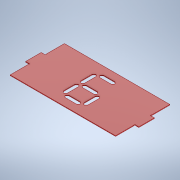
# Autodesk Inventor part: Cockpit_front_frame_cloth
Saved by Autodesk Inventor 2020.4 (Build 244396000, 396)
## iProperties
Created: 2022-04-01
Part Number: Cockpit_front_frame_cloth
Material: 一般
Document SubType Name: Modeling
Designer: Masato Kubotera
Density: 1 g/cm^3
Appearance: 滑らか - 赤
Author: Masato Kubotera
Autodesk Inventor part; units mm, degrees
ref_plane "XZ Plane" through (0, 0, 0) normal (0, 1, 0) x (-1, 0, 0)
ref_plane "XY Plane" through (0, 0, 0) normal (0, 0, 1) x (1, 0, 0)
derived "Cockpit_front_frame.ipt"
sketch "スケッチ2" plane through (0, 0, 0) normal (0, 1, 0) x (-1, 0, 0)
  line L0 (-28.5, -22.5) -> (88.5, -22.5) construction
  line L1 (88.5, -22.5) -> (88.5, -138.5)
  line L2 (88.5, -96) -> (-28.5, -96) construction
  line L3 (-28.5, -96) -> (-28.5, -22.5) construction
  line L4 (-28.5, -22.5) -> (88.5, -96) construction
  line L5 (88.5, -22.5) -> (-28.5, -96) construction
  line L6 (38.5, -101) -> (38.5, -133.5)
  line L7 (43.5, -138.5) -> (88.5, -138.5)
  line L8 (63.9, -63.85) -> (73.1, -63.85) construction
  line L9 (73.1, -63.85) -> (73.1, -77.65) construction
  line L10 (73.1, -77.65) -> (63.9, -77.65) construction
  line L11 (63.9, -77.65) -> (63.9, -63.85) construction
  line L12 (63.9, -63.85) -> (73.1, -77.65) construction
  line L13 (73.1, -63.85) -> (63.9, -77.65) construction
  line L14 (63.2, -63.2) -> (73.8, -63.2) construction
  line L15 (73.8, -63.2) -> (73.8, -78.3) construction
  line L16 (73.8, -78.3) -> (63.2, -78.3) construction
  line L17 (63.2, -78.3) -> (63.2, -63.2) construction
  line L18 (63.2, -63.2) -> (73.8, -78.3) construction
  line L19 (73.8, -63.2) -> (63.2, -78.3) construction
  line L20 (68.5, -63.2) -> (68.5, -78.3) construction
  line L21 (73.8, -70.75) -> (63.2, -70.75) construction
  line L22 (64.6349, -63.15) -> (72.3651, -63.15)
  line L23 (63.15, -64.6349) -> (63.15, -76.8651)
  line L24 (65.3349, -63.8) -> (71.6651, -63.8)
  line L25 (63.85, -65.2849) -> (63.85, -76.2151)
  arc A0 (64.6349, -63.15) -> (63.15, -64.6349) centre (63.8925, -63.8925) ccw
  arc A1 (65.3349, -63.8) -> (63.85, -65.2849) centre (64.5925, -64.5425) ccw
  arc A2 (73.85, -64.6349) -> (72.3651, -63.15) centre (73.1075, -63.8925) ccw
  arc A3 (73.15, -65.2849) -> (71.6651, -63.8) centre (72.4075, -64.5425) ccw
  line L26 (64.6349, -78.35) -> (72.3651, -78.35)
  line L27 (65.3349, -77.7) -> (71.6651, -77.7)
  arc A4 (63.85, -76.2151) -> (65.3349, -77.7) centre (64.5925, -76.9575) ccw
  arc A5 (63.15, -76.8651) -> (64.6349, -78.35) centre (63.8925, -77.6075) ccw
  arc A6 (72.3651, -78.35) -> (73.85, -76.8651) centre (73.1075, -77.6075) ccw
  arc A7 (71.6651, -77.7) -> (73.15, -76.2151) centre (72.4075, -76.9575) ccw
  line L28 (73.15, -65.2849) -> (73.15, -76.2151)
  line L29 (73.85, -64.6349) -> (73.85, -76.8651)
  line L30 (-23.5, -22.5) -> (-28.5, -27.5)
  line L31 (-28.5, -59.25) -> (88.5, -59.25) construction
  line L32 (30, -22.5) -> (30, -96) construction
  line L33 (-23.5, -96) -> (-28.5, -91)
  line L34 (-28.5, -27.5) -> (-28.5, -91)
  line L35 (-20.5, -24.5) -> (-25.5, -24.5) construction
  line L36 (-25.5, -24.5) -> (-25.5, -94) construction
  line L37 (-25.5, -94) -> (-20.5, -94) construction
  line L38 (-20.5, -94) -> (-20.5, -24.5) construction
  line L39 (-20.5, -24.5) -> (-25.5, -94) construction
  line L40 (-25.5, -24.5) -> (-20.5, -94) construction
  line L41 (-25.55, -46.7) -> (-20.45, -46.7)
  line L42 (-20.45, -46.7) -> (-20.45, -71.8)
  line L43 (-20.45, -71.8) -> (-25.55, -71.8)
  line L44 (-25.55, -71.8) -> (-25.55, -46.7)
  line L45 (-25.55, -46.7) -> (-20.45, -71.8) construction
  line L46 (-20.45, -46.7) -> (-25.55, -71.8) construction
  line L47 (-25.5, -46.75) -> (-20.5, -46.75) construction
  line L48 (-25.5, -71.75) -> (-20.5, -71.75) construction
  line L49 (-23, -24.5) -> (-23, -94) construction
  circle A8 centre (-23, -35) radius 3
  circle A9 centre (-23, -35) radius 1.6
  arc A10 (-24.0651, -46.7) -> (-25.55, -48.1849) centre (-24.8075, -47.4425) ccw
  arc A11 (-20.45, -48.1849) -> (-21.9349, -46.7) centre (-21.1925, -47.4425) ccw
  arc A12 (-25.55, -70.3151) -> (-24.0651, -71.8) centre (-24.8075, -71.0575) ccw
  arc A13 (-21.9349, -71.8) -> (-20.45, -70.3151) centre (-21.1925, -71.0575) ccw
  circle A14 centre (-23, -83.5) radius 3
  circle A15 centre (-23, -83.5) radius 1.6
  line L50 (33.5, -96) -> (38.5, -101)
  line L51 (-23.5, -96) -> (33.5, -96)
  line L52 (81, -46.5) -> (-20.5, -46.5) construction
  line L53 (-20.5, -46.5) -> (-20.5, -41.5) construction
  line L54 (-20.5, -41.5) -> (81, -41.5) construction
  line L55 (81, -41.5) -> (81, -46.5) construction
  line L56 (81, -46.5) -> (-20.5, -41.5) construction
  line L57 (-20.5, -46.5) -> (81, -41.5) construction
  line L58 (-20.5, -44) -> (81, -44) construction
  line L59 (30.25, -41.5) -> (30.25, -46.5) construction
  line L60 (5.25, -41.5) -> (5.25, -46.5) construction
  line L61 (55.3, -41.45) -> (5.2, -41.45)
  line L62 (5.2, -41.45) -> (5.2, -46.55)
  line L63 (5.2, -46.55) -> (55.3, -46.55)
  line L64 (55.3, -46.55) -> (55.3, -41.45)
  line L65 (55.3, -41.45) -> (5.2, -46.55) construction
  line L66 (5.2, -41.45) -> (55.3, -46.55) construction
  arc A16 (6.6849, -41.45) -> (5.2, -42.9349) centre (5.9425, -42.1925) ccw
  circle A17 centre (-2.25, -44) radius 3
  circle A18 centre (-2.25, -44) radius 1.6
  line L67 (55.25, -41.5) -> (55.25, -46.5) construction
  arc A19 (55.3, -42.9349) -> (53.8151, -41.45) centre (54.5575, -42.1925) ccw
  circle A20 centre (62.75, -44) radius 3
  circle A21 centre (62.75, -44) radius 1.6
  arc A22 (5.2, -45.0651) -> (6.6849, -46.55) centre (5.9425, -45.8075) ccw
  arc A23 (53.8151, -46.55) -> (55.3, -45.0651) centre (54.5575, -45.8075) ccw
  line L68 (-20.5, -89) -> (81, -89) construction
  line L69 (81, -89) -> (81, -94) construction
  line L70 (81, -94) -> (-20.5, -94) construction
  line L71 (-20.5, -94) -> (-20.5, -89) construction
  line L72 (-20.5, -89) -> (81, -94) construction
  line L73 (81, -89) -> (-20.5, -94) construction
  line L74 (-20.5, -91.5) -> (81, -91.5) construction
  line L75 (30.25, -89) -> (30.25, -94) construction
  line L76 (55.3, -91.55) -> (5.2, -91.55)
  line L77 (5.2, -91.55) -> (5.2, -88.95)
  line L78 (5.2, -88.95) -> (55.3, -88.95)
  line L79 (55.3, -88.95) -> (55.3, -91.55)
  line L80 (55.3, -91.55) -> (5.2, -88.95) construction
  line L81 (5.2, -91.55) -> (55.3, -88.95) construction
  line L82 (5.25, -89) -> (5.25, -91.5) construction
  line L83 (55.25, -89) -> (55.25, -91.5) construction
  line L84 (5.25, -90.25) -> (55.25, -90.25) construction
  arc A24 (7.3, -88.95) -> (5.2, -88.95) centre (6.25, -88.95) ccw
  arc A25 (55.3, -88.95) -> (53.2, -88.95) centre (54.25, -88.95) ccw
  arc A26 (5.2, -91.55) -> (7.3, -91.55) centre (6.25, -91.55) ccw
  arc A27 (53.2, -91.55) -> (55.3, -91.55) centre (54.25, -91.55) ccw
  circle A28 centre (-2.5, -91.5) radius 3
  circle A29 centre (-2.5, -91.5) radius 1.6
  circle A30 centre (62.5, -91.5) radius 3 construction
  circle A31 centre (62.5, -91.5) radius 1.6 construction
  line L85 (-23.5, -22.5) -> (63.7651, -22.5)
  line L86 (65.25, -21.0151) -> (65.25, -17.5)
  line L87 (65.25, -17.5) -> (73.25, -17.5)
  line L88 (73.25, -17.5) -> (73.25, -21.0151)
  line L89 (81, -22.5) -> (81, -17.5)
  line L90 (88.5, -22.5) -> (88.5, -20)
  line L91 (81, -17.5) -> (86, -17.5)
  line L92 (86, -17.5) -> (88.5, -20)
  line L93 (69.25, -17.5) -> (69.25, -22.5) construction
  arc A32 (63.7651, -22.5) -> (65.25, -21.0151) centre (64.5075, -21.7575) ccw
  arc A33 (73.25, -21.0151) -> (74.7349, -22.5) centre (73.9925, -21.7575) ccw
  arc A34 (79.5151, -22.5) -> (81, -21.0151) centre (80.2575, -21.7575) ccw
  line L94 (-15.5, -89) -> (-15.5, -69) construction
  line L95 (-15.5, -69) -> (64.5, -69) construction
  line L96 (64.5, -69) -> (64.5, -89) construction
  line L97 (45.5, -84) -> (-16.5, -84)
  line L98 (-18.5, -82) -> (-18.5, -63.3955)
  line L99 (-16.5, -61.3955) -> (45.5, -61.3955)
  line L100 (47.5, -63.3955) -> (47.5, -82)
  line L101 (47.5, -84) -> (-18.5, -61.3955) construction
  line L102 (-18.5, -84) -> (47.5, -61.3955) construction
  arc A35 (-16.5, -61.3955) -> (-18.5, -63.3955) centre (-16.5, -63.3955) ccw
  arc A36 (-18.5, -82) -> (-16.5, -84) centre (-16.5, -82) ccw
  arc A37 (45.5, -84) -> (47.5, -82) centre (45.5, -82) ccw
  arc A38 (47.5, -63.3955) -> (45.5, -61.3955) centre (45.5, -63.3955) ccw
  line L103 (38.5, -133.5) -> (43.5, -138.5)
  line L104 (46, -131) -> (41, -131) construction
  line L105 (41, -131) -> (41, -96) construction
  line L106 (41, -96) -> (46, -96) construction
  line L107 (46, -96) -> (46, -131) construction
  line L108 (46, -131) -> (41, -96) construction
  line L109 (41, -131) -> (46, -96) construction
  line L110 (43.5, -96) -> (43.5, -131) construction
  line L111 (41, -113.5) -> (46, -113.5) construction
  line L112 (43.5, -107.5) -> (46, -107.5) construction
  line L113 (43.45, -107.45) -> (46.05, -107.45)
  line L114 (46.05, -107.45) -> (46.05, -119.55)
  line L115 (46.05, -119.55) -> (43.45, -119.55)
  line L116 (43.45, -119.55) -> (43.45, -107.45)
  line L117 (43.45, -107.45) -> (46.05, -119.55) construction
  line L118 (46.05, -107.45) -> (43.45, -119.55) construction
  arc A39 (46.05, -109.55) -> (46.05, -107.45) centre (46.05, -108.5) ccw
  arc A40 (44.9349, -107.45) -> (43.45, -108.9349) centre (44.1925, -108.1925) ccw
  line L119 (43.5, -119.5) -> (46, -119.5) construction
  arc A41 (46.05, -119.55) -> (46.05, -117.45) centre (46.05, -118.5) ccw
  arc A42 (43.45, -118.0651) -> (44.9349, -119.55) centre (44.1925, -118.8075) ccw
  line L120 (44.75, -107.5) -> (44.75, -119.5) construction
  circle A43 centre (43.5, -125.5) radius 3 construction
  circle A44 centre (43.5, -125.5) radius 1.6 construction
  circle A45 centre (43.5, -101.5) radius 3
  circle A46 centre (43.5, -101.5) radius 1.6
  circle A47 centre (-13.5, -55) radius 2
  line L121 (41, -131) -> (79.8645, -131) construction
  line L122 (79.8645, -131) -> (79.8645, -136) construction
  line L123 (79.8645, -136) -> (41, -136) construction
  line L124 (41, -136) -> (41, -131) construction
  line L125 (41, -131) -> (79.8645, -136) construction
  line L126 (79.8645, -131) -> (41, -136) construction
  line L127 (41, -133.5) -> (79.8645, -133.5) construction
  line L128 (60.4322, -131) -> (60.4322, -136) construction
  line L129 (60.4322, -133.5) -> (60.4322, -131) construction
  line L130 (52.8822, -130.95) -> (67.9822, -130.95)
  line L131 (67.9822, -130.95) -> (67.9822, -133.55)
  line L132 (67.9822, -133.55) -> (52.8822, -133.55)
  line L133 (52.8822, -133.55) -> (52.8822, -130.95)
  line L134 (52.8822, -130.95) -> (67.9822, -133.55) construction
  line L135 (67.9822, -130.95) -> (52.8822, -133.55) construction
  line L136 (52.9322, -131) -> (52.9322, -133.5) construction
  arc A48 (54.9822, -130.95) -> (52.8822, -130.95) centre (53.9322, -130.95) ccw
  arc A49 (52.8822, -132.0651) -> (54.3672, -133.55) centre (53.6247, -132.8075) ccw
  arc A50 (67.9822, -130.95) -> (65.8822, -130.95) centre (66.9322, -130.95) ccw
  arc A51 (66.4973, -133.55) -> (67.9822, -132.0651) centre (67.2398, -132.8075) ccw
  line L137 (67.9322, -131) -> (67.9322, -133.5) construction
  line L138 (52.9322, -132.25) -> (67.9322, -132.25) construction
  circle A52 centre (74.4322, -133.5) radius 1.6 construction
  circle A53 centre (74.4322, -133.5) radius 3 construction
  circle A54 centre (46.4322, -133.5) radius 1.6
  circle A55 centre (46.4322, -133.5) radius 3
  line L139 (50.5, -96.5) -> (79, -96.5)
  line L140 (81, -98.5) -> (81, -126.5)
  line L141 (79, -128.5) -> (50.5, -128.5)
  line L142 (48.5, -126.5) -> (48.5, -98.5)
  line L143 (48.5, -96.5) -> (81, -128.5) construction
  line L144 (81, -96.5) -> (48.5, -128.5) construction
  arc A56 (50.5, -96.5) -> (48.5, -98.5) centre (50.5, -98.5) ccw
  arc A57 (48.5, -126.5) -> (50.5, -128.5) centre (50.5, -126.5) ccw
  arc A58 (79, -128.5) -> (81, -126.5) centre (79, -126.5) ccw
  arc A59 (81, -98.5) -> (79, -96.5) centre (79, -98.5) ccw
  line L145 (81, -91.6746) -> (86, -91.6746) construction
  line L146 (86, -91.6746) -> (86, -136) construction
  line L147 (86, -136) -> (81, -136) construction
  line L148 (81, -136) -> (81, -91.6746) construction
  line L149 (81, -91.6746) -> (86, -136) construction
  line L150 (86, -91.6746) -> (81, -136) construction
  line L151 (83.5, -91.6746) -> (83.5, -136) construction
  circle A60 centre (83.5, -94.1746) radius 1.475
  circle A61 centre (83.5, -99.1746) radius 1.475
  circle A62 centre (83.5, -104.1746) radius 1.475
  circle A63 centre (83.5, -133.5) radius 1.6
  arc A64 (86, -91.6746) -> (81, -91.6746) centre (83.5, -133.5) ccw construction
  arc A65 (86.0112, -91.5751) -> (80.9888, -91.5751) centre (83.5, -133.5) ccw construction
  line L152 (88.5, -133.5) -> (83.5, -138.5)
  arc A66 (81, -131) -> (86, -136) centre (83.5, -133.5) ccw construction
  line L153 (86, -91.5) -> (81, -91.5) construction
  circle A67 centre (83.5, -133.5) radius 3
  line L154 (77.125, -22.5) -> (77.125, -27.147) construction
  line L155 (61.375, -22.5) -> (61.375, -27.147) construction
  line L156 (65.25, -22.5) -> (73.25, -22.5)
  line L157 (-18.5, -29.5) -> (-18.5, -34.7517)
  line L158 (-16.5, -36.7517) -> (45.5, -36.7517)
  line L159 (47.5, -34.7517) -> (47.5, -29.5)
  line L160 (45.5, -27.5) -> (-16.5, -27.5)
  arc A68 (-16.5, -27.5) -> (-18.5, -29.5) centre (-16.5, -29.5) ccw
  arc A69 (-18.5, -34.7517) -> (-16.5, -36.7517) centre (-16.5, -34.7517) ccw
  arc A70 (45.5, -36.7517) -> (47.5, -34.7517) centre (45.5, -34.7517) ccw
  arc A71 (47.5, -29.5) -> (45.5, -27.5) centre (45.5, -29.5) ccw
  line L161 (81, -66.9105) -> (86, -66.9105) construction
  line L162 (86, -66.9105) -> (86, -46.9105) construction
  line L163 (86, -46.9105) -> (81, -46.9105) construction
  line L164 (81, -46.9105) -> (81, -66.9105) construction
  line L165 (81, -66.9105) -> (86, -46.9105) construction
  line L166 (86, -66.9105) -> (81, -46.9105) construction
  line L167 (81, -22.5) -> (81, -28.5) construction
  line L168 (81, -28.5) -> (57.5, -28.5) construction
  line L169 (57.5, -28.5) -> (57.5, -22.5) construction
  line L170 (74.7349, -22.5) -> (79.5151, -22.5) construction
  line L171 (74.7349, -22.5) -> (79.5151, -22.5)
  point P0 (0, 0)
  point P1 (30, -59.25)
  point P2 (-25.7227, -96)
  point P3 (68.5, -70.75)
  point P4 (63.15, -63.15)
  point P5 (63.85, -63.8)
  point P6 (-23, -59.25)
  point P7 (30.25, -44)
  point P8 (30.25, -91.5)
  point P9 (30.25, -90.25)
  point P10 (30.25, -90.25)
  point P11 (52.5, -22)
  point P12 (14.5, -72.6978)
  point P13 (-18.5, -61)
  point P14 (47.5, -61)
  point P15 (43.5, -113.5)
  point P16 (44.75, -113.5)
  point P17 (60.4322, -132.25)
  point P18 (64.75, -112.5)
  point P19 (83.5, -113.8373)
  point P20 (-18.5, -36.7517)
  point P21 (47.5, -27.5)
  point P22 (-18.5, -27.5)
  point P23 (83.5, -56.9105)
  point P24 (69.25, -28.5)
sketch "スケッチ3" plane through (20.5, 0, 0) normal (1, 0, 0) x (0, 1, 0)
  line L0 (-135, -24.5) -> (0, -24.5)
  line L1 (0, -24.5) -> (0, -94)
  line L2 (0, -94) -> (-135, -94)
  line L3 (-135, -94) -> (-135, -24.5)
  line L4 (-135, -24.5) -> (0, -94) construction
  line L5 (0, -24.5) -> (-135, -94) construction
  line L6 (0, -71.75) -> (5, -71.75)
  line L7 (5, -71.75) -> (5, -46.75)
  line L8 (5, -46.75) -> (0, -46.75)
  line L9 (0, -59.25) -> (-135, -59.25) construction
  line L10 (-67.5, -94) -> (-67.5, -24.5)
  arc A0 (1.4849, -71.75) -> (0, -73.2349) centre (0.7425, -72.4925) ccw
  arc A1 (0, -45.2651) -> (1.4849, -46.75) centre (0.7425, -46.0075) ccw
  line L11 (-128, -89) -> (-7, -89)
  line L12 (-5, -87) -> (-5, -48.5)
  line L13 (-7, -46.5) -> (-128, -46.5)
  line L14 (-130, -48.5) -> (-130, -87)
  line L15 (-130, -89) -> (-5, -46.5) construction
  line L16 (-5, -89) -> (-130, -46.5) construction
  line L17 (-128, -29.5) -> (-7, -29.5)
  line L18 (-5, -31.5) -> (-5, -39.5)
  line L19 (-7, -41.5) -> (-128, -41.5)
  line L20 (-130, -39.5) -> (-130, -31.5)
  line L21 (-130, -29.5) -> (-5, -41.5) construction
  line L22 (-5, -29.5) -> (-130, -41.5) construction
  arc A2 (-7, -89) -> (-5, -87) centre (-7, -87) ccw
  arc A3 (-5, -48.5) -> (-7, -46.5) centre (-7, -48.5) ccw
  arc A4 (-128, -46.5) -> (-130, -48.5) centre (-128, -48.5) ccw
  arc A5 (-130, -87) -> (-128, -89) centre (-128, -87) ccw
  arc A6 (-130, -39.5) -> (-128, -41.5) centre (-128, -39.5) ccw
  arc A7 (-7, -41.5) -> (-5, -39.5) centre (-7, -39.5) ccw
  arc A8 (-5, -31.5) -> (-7, -29.5) centre (-7, -31.5) ccw
  arc A9 (-128, -29.5) -> (-130, -31.5) centre (-128, -31.5) ccw
  point P0 (0, 0)
  point P1 (-67.5, -59.25)
  point P2 (0, -24.5)
  point P3 (0, -46.5)
  point P4 (0, -46.5)
  point P5 (0, -46.5)
  point P6 (0, -41.5)
  point P7 (0, -41.5)
  point P8 (0, -41.5)
  point P9 (-67.5, -67.75)
  point P10 (-67.5, -35.5)
ref_plane "作業平面1" through (10, 0, 0) normal (1, 0, 0) x (0, 1, 0)
sketch "スケッチ4" plane through (10, 0, 0) normal (1, 0, 0) x (0, 1, 0)
  line L0 (-135, -24.5) -> (0, -24.5)
  line L1 (0, -24.5) -> (0, -94)
  line L2 (0, -94) -> (-135, -94)
  line L3 (-135, -94) -> (-135, -24.5)
  line L4 (0, -49.25) -> (5, -49.25)
  line L5 (5, -49.25) -> (5, -69.25)
  line L6 (5, -69.25) -> (0, -69.25)
  arc A0 (0, -47.7651) -> (1.4849, -49.25) centre (0.7425, -48.5075) ccw
  line L7 (5, -71.75) -> (5, -46.75) projected
  line L8 (0, -59.25) -> (-135, -59.25) construction
  arc A1 (1.4849, -69.25) -> (0, -70.7349) centre (0.7425, -69.9925) ccw
  line L9 (-67.5, -94) -> (-67.5, -24.5) construction
  line L10 (-135, -49.25) -> (-140, -49.25)
  line L11 (-140, -49.25) -> (-140, -69.25)
  line L12 (-140, -69.25) -> (-135, -69.25)
  arc A2 (-136.4849, -49.25) -> (-135, -47.7651) centre (-135.7425, -48.5075) ccw
  arc A3 (-135, -70.7349) -> (-136.4849, -69.25) centre (-135.7425, -69.9925) ccw
  line L13 (-74.5858, -61.75) -> (-60.4142, -61.75)
  line L14 (-60, -61.75) -> (-60, -56.75) construction
  line L15 (-60.4142, -56.75) -> (-74.5858, -56.75)
  line L16 (-75, -56.75) -> (-75, -61.75) construction
  line L17 (-75, -61.75) -> (-60, -56.75) construction
  line L18 (-60, -61.75) -> (-75, -56.75) construction
  line L19 (-75.2929, -57.0429) -> (-76.7929, -58.5429)
  line L20 (-76.7929, -59.9571) -> (-75.2929, -61.4571)
  line L21 (-59.7071, -57.0429) -> (-58.2071, -58.5429)
  line L22 (-58.2071, -59.9571) -> (-59.7071, -61.4571)
  line L23 (-83.1569, -40.6642) -> (-78.1569, -40.6642) construction
  line L24 (-78.1569, -41.0784) -> (-78.1569, -55.25)
  line L25 (-78.1569, -55.6642) -> (-83.1569, -55.6642) construction
  line L26 (-83.1569, -55.25) -> (-83.1569, -41.0784)
  line L27 (-83.1569, -40.6642) -> (-78.1569, -55.6642) construction
  line L28 (-78.1569, -40.6642) -> (-83.1569, -55.6642) construction
  line L29 (-82.864, -55.9571) -> (-81.364, -57.4571)
  line L30 (-79.9497, -57.4571) -> (-78.4497, -55.9571)
  line L31 (-82.864, -40.3713) -> (-81.364, -38.8713)
  line L32 (-79.9497, -38.8713) -> (-78.4497, -40.3713)
  arc A4 (-76.7929, -58.5429) -> (-76.7929, -59.9571) centre (-76.0858, -59.25) ccw
  arc A5 (-74.5858, -56.75) -> (-75.2929, -57.0429) centre (-74.5858, -57.75) ccw
  arc A6 (-75.2929, -61.4571) -> (-74.5858, -61.75) centre (-74.5858, -60.75) ccw
  arc A7 (-60.4142, -61.75) -> (-59.7071, -61.4571) centre (-60.4142, -60.75) ccw
  arc A8 (-58.2071, -59.9571) -> (-58.2071, -58.5429) centre (-58.9142, -59.25) ccw
  arc A9 (-59.7071, -57.0429) -> (-60.4142, -56.75) centre (-60.4142, -57.75) ccw
  arc A10 (-81.364, -57.4571) -> (-79.9497, -57.4571) centre (-80.6569, -56.75) ccw
  arc A11 (-83.1569, -55.25) -> (-82.864, -55.9571) centre (-82.1569, -55.25) ccw
  arc A12 (-78.4497, -55.9571) -> (-78.1569, -55.25) centre (-79.1569, -55.25) ccw
  arc A13 (-82.864, -40.3713) -> (-83.1569, -41.0784) centre (-82.1569, -41.0784) ccw
  arc A14 (-79.9497, -38.8713) -> (-81.364, -38.8713) centre (-80.6569, -39.5784) ccw
  arc A15 (-78.1569, -41.0784) -> (-78.4497, -40.3713) centre (-79.1569, -41.0784) ccw
  line L33 (-53.636, -57.4571) -> (-52.136, -55.9571)
  arc A16 (-55.0503, -57.4571) -> (-53.636, -57.4571) centre (-54.3431, -56.75) ccw
  line L34 (-56.5503, -55.9571) -> (-55.0503, -57.4571)
  arc A17 (-56.8431, -55.25) -> (-56.5503, -55.9571) centre (-55.8431, -55.25) ccw
  line L35 (-56.8431, -55.25) -> (-56.8431, -41.0784)
  arc A18 (-52.136, -55.9571) -> (-51.8431, -55.25) centre (-52.8431, -55.25) ccw
  line L36 (-51.8431, -41.0784) -> (-51.8431, -55.25)
  line L37 (-56.5503, -40.3713) -> (-55.0503, -38.8713)
  arc A19 (-56.5503, -40.3713) -> (-56.8431, -41.0784) centre (-55.8431, -41.0784) ccw
  arc A20 (-53.636, -38.8713) -> (-55.0503, -38.8713) centre (-54.3431, -39.5784) ccw
  line L38 (-53.636, -38.8713) -> (-52.136, -40.3713)
  arc A21 (-51.8431, -41.0784) -> (-52.136, -40.3713) centre (-52.8431, -41.0784) ccw
  line L39 (-79.9497, -79.6287) -> (-78.4497, -78.1287)
  arc A22 (-81.364, -79.6287) -> (-79.9497, -79.6287) centre (-80.6569, -78.9216) ccw
  line L40 (-82.864, -78.1287) -> (-81.364, -79.6287)
  arc A23 (-83.1569, -77.4216) -> (-82.864, -78.1287) centre (-82.1569, -77.4216) ccw
  line L41 (-83.1569, -77.4216) -> (-83.1569, -63.25)
  arc A24 (-78.4497, -78.1287) -> (-78.1569, -77.4216) centre (-79.1569, -77.4216) ccw
  line L42 (-78.1569, -63.25) -> (-78.1569, -77.4216)
  line L43 (-82.864, -62.5429) -> (-81.364, -61.0429)
  arc A25 (-82.864, -62.5429) -> (-83.1569, -63.25) centre (-82.1569, -63.25) ccw
  arc A26 (-79.9497, -61.0429) -> (-81.364, -61.0429) centre (-80.6569, -61.75) ccw
  line L44 (-79.9497, -61.0429) -> (-78.4497, -62.5429)
  arc A27 (-78.1569, -63.25) -> (-78.4497, -62.5429) centre (-79.1569, -63.25) ccw
  line L45 (-53.636, -79.6287) -> (-52.136, -78.1287)
  arc A28 (-55.0503, -79.6287) -> (-53.636, -79.6287) centre (-54.3431, -78.9216) ccw
  line L46 (-56.5503, -78.1287) -> (-55.0503, -79.6287)
  arc A29 (-56.8431, -77.4216) -> (-56.5503, -78.1287) centre (-55.8431, -77.4216) ccw
  line L47 (-56.8431, -77.4216) -> (-56.8431, -63.25)
  arc A30 (-52.136, -78.1287) -> (-51.8431, -77.4216) centre (-52.8431, -77.4216) ccw
  line L48 (-51.8431, -63.25) -> (-51.8431, -77.4216)
  line L49 (-56.5503, -62.5429) -> (-55.0503, -61.0429)
  arc A31 (-56.5503, -62.5429) -> (-56.8431, -63.25) centre (-55.8431, -63.25) ccw
  arc A32 (-53.636, -61.0429) -> (-55.0503, -61.0429) centre (-54.3431, -61.75) ccw
  line L50 (-53.636, -61.0429) -> (-52.136, -62.5429)
  arc A33 (-51.8431, -63.25) -> (-52.136, -62.5429) centre (-52.8431, -63.25) ccw
  line L51 (-74.5858, -39.5784) -> (-60.4142, -39.5784)
  arc A34 (-75.2929, -39.2855) -> (-74.5858, -39.5784) centre (-74.5858, -38.5784) ccw
  line L52 (-76.7929, -37.7855) -> (-75.2929, -39.2855)
  arc A35 (-76.7929, -36.3713) -> (-76.7929, -37.7855) centre (-76.0858, -37.0784) ccw
  arc A36 (-74.5858, -34.5784) -> (-75.2929, -34.8713) centre (-74.5858, -35.5784) ccw
  line L53 (-60.4142, -34.5784) -> (-74.5858, -34.5784)
  line L54 (-75.2929, -34.8713) -> (-76.7929, -36.3713)
  arc A37 (-59.7071, -34.8713) -> (-60.4142, -34.5784) centre (-60.4142, -35.5784) ccw
  line L55 (-59.7071, -34.8713) -> (-58.2071, -36.3713)
  arc A38 (-58.2071, -37.7855) -> (-58.2071, -36.3713) centre (-58.9142, -37.0784) ccw
  line L56 (-58.2071, -37.7855) -> (-59.7071, -39.2855)
  arc A39 (-60.4142, -39.5784) -> (-59.7071, -39.2855) centre (-60.4142, -38.5784) ccw
  arc A40 (-74.5858, -78.9216) -> (-75.2929, -79.2145) centre (-74.5858, -79.9216) ccw
  line L57 (-75.2929, -79.2145) -> (-76.7929, -80.7145)
  arc A41 (-76.7929, -80.7145) -> (-76.7929, -82.1287) centre (-76.0858, -81.4216) ccw
  line L58 (-76.7929, -82.1287) -> (-75.2929, -83.6287)
  arc A42 (-75.2929, -83.6287) -> (-74.5858, -83.9216) centre (-74.5858, -82.9216) ccw
  line L59 (-74.5858, -83.9216) -> (-60.4142, -83.9216)
  arc A43 (-60.4142, -83.9216) -> (-59.7071, -83.6287) centre (-60.4142, -82.9216) ccw
  line L60 (-58.2071, -82.1287) -> (-59.7071, -83.6287)
  arc A44 (-58.2071, -82.1287) -> (-58.2071, -80.7145) centre (-58.9142, -81.4216) ccw
  line L61 (-59.7071, -79.2145) -> (-58.2071, -80.7145)
  arc A45 (-59.7071, -79.2145) -> (-60.4142, -78.9216) centre (-60.4142, -79.9216) ccw
  line L62 (-60.4142, -78.9216) -> (-74.5858, -78.9216)
  point P0 (0, 0)
  point P1 (1.4849, -69.25)
  point P2 (-135, -47.7651)
  point P3 (0, -70.7349)
  point P4 (-67.5, -59.25)
  point P5 (-67.5, -59.25)
  point P6 (-80.6569, -48.1642)
  point P7 (-51.8431, -55.6642)
  point P8 (-56.8431, -55.6642)
  point P9 (-56.8431, -40.6642)
  point P10 (-51.8431, -40.6642)
  point P11 (-78.1569, -77.8358)
  point P12 (-83.1569, -77.8358)
  point P13 (-83.1569, -62.8358)
  point P14 (-78.1569, -62.8358)
  point P15 (-51.8431, -77.8358)
  point P16 (-56.8431, -77.8358)
  point P17 (-56.8431, -62.8358)
  point P18 (-51.8431, -62.8358)
  point P19 (-75, -39.5784)
  point P20 (-60, -39.5784)
  point P21 (-75, -34.5784)
  point P22 (-60, -34.5784)
  point P23 (-75, -78.9216)
  point P24 (-75, -83.9216)
  point P25 (-60, -83.9216)
  point P26 (-60, -78.9216)
  point P27 (-135, -49.25)
  point P28 (0, -69.25)
  dimension "d2" = 1.05
  dimension "d3" = 20
  dimension "d7" = 5
  dimension "d8" = 15
  dimension "d9" = 15
  dimension "d10" = 5
  dimension "d11" = 1
  dimension "d14" = 26.3137
  dimension "d17" = 22.1716
  dimension "d20" = 3
  dimension "d21" = 3
  dimension "d22" = 3
  dimension "d25" = 22.1716
  dimension "d30" = 3
  dimension "d31" = 3
  dimension "d34" = 22.1716
  dimension "d39" = 3
  constraints: 120 end point, 93 point on circle, 61 point on line, 46 centre point, 24 tangent, 13 symmetric about line, 11 equal radius, 10 parallel, 8 perpendicular, 7 midpoint, 5 horizontal, 3 vertical, 2 coincident, 1 collinear, 176 other
  measures "d2" radius of A0
  measures "d3" distance of L4.end L5.end
  measures "d7" distance of L14.start L14.end
  measures "d8" distance of L16.end L14.start
  measures "d9" distance of L23.end L25.start
  measures "d10" distance of L23.start L23.end
  measures "d11" radius of A4
  measures "d14" distance of L30.start L33.start
  measures "d17" distance of L30.start L39.start
  measures "d20" distance between parallel lines of L30 L19
  measures "d21" distance between parallel lines of L34 L21
  measures "d22" distance between parallel lines of L20 L44
  measures "d25" distance of L13.start L51.start
  measures "d30" distance between parallel lines of L32 L52
  measures "d34" distance of A5.centre A40.centre
  measures "d39" distance between parallel lines of L39 L57
extrude "押し出し1" add sketch "スケッチ4" along normal blind 0.75 contours L0 L1 A0 A1 L2 L3 A3 A2 | L3 A3 L12 L11 L10 A2 | A0 L4 L5 L6 A1 L1 | A16 L34 A17 L35 A19 L37 A20 L38 A21 L36 A18 L33
equation "\"d9\" = d8"
equation "\"d10\" = d7"
equation "\"d21\" = d20"
equation "\"d22\" = d20"
equation "\"d30\" = d20"
equation "\"d31\" = d20"
equation "\"d39\" = d20"
